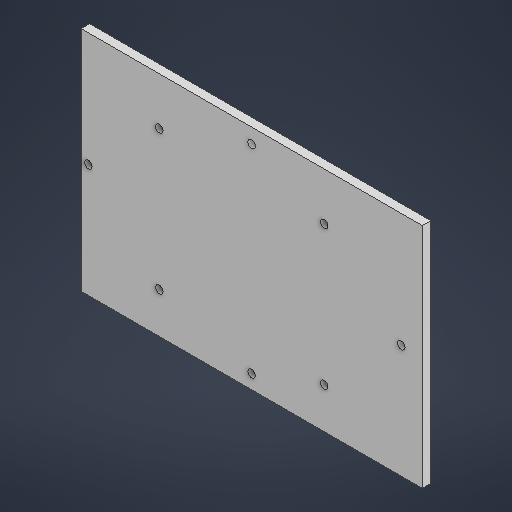
# Autodesk Inventor part: plate
Saved by Autodesk Inventor 2026.1 (Build 301233020, 233B)
## iProperties
Created: 2026-01-14
Part Number: plate
Material: Generic
Document SubType Name: Modeling
Designer: osama
Density: 1 g/cm^3
Appearance: Default
Author: osama
Autodesk Inventor part; units mm, degrees
ref_plane "YZ Plane" through (0, 0, 0) normal (1, 0, 0) x (0, 1, 0)
ref_plane "XZ Plane" through (0, 0, 0) normal (0, 1, 0) x (-1, 0, 0)
ref_plane "XY Plane" through (0, 0, 0) normal (0, 0, 1) x (1, 0, 0)
sketch "Sketch1" plane through (0, 0, 0) normal (0, 0, 1) x (1, 0, 0)
  line L0 (-60, -40) -> (60, -40)
  line L1 (60, -40) -> (60, 40)
  line L2 (60, 40) -> (-60, 40)
  line L3 (-60, 40) -> (-60, -40)
  line L4 (-60, -40) -> (60, 40) construction
  line L5 (60, -40) -> (-60, 40) construction
  line L6 (60, 0) -> (-60, 0)
  line L7 (0, -40) -> (0, 40)
  point P0 (0, 0)
  dimension "d0" = 120
  dimension "d1" = 80
  constraints: 16 end point, 6 midpoint, 2 parallel, 1 horizontal, 1 perpendicular
  measures "d0" distance of L2.end L1.end
  measures "d1" distance of L1.end L0.end
extrude "Extrusion1" add sketch "Sketch1" along normal blind 3
sketch "Sketch2" plane through (0, 0, 3) normal (0, 0, 1) x (1, 0, 0)
  circle A0 centre (-0.0328, 34.8037) radius 1.35
  circle A1 centre (-0.0328, -35.0463) radius 1.35
  circle A2 centre (52.5922, -0.1213) radius 1.35
  circle A3 centre (25.4936, 23.3086) radius 1.35
  circle A4 centre (25.4936, -25.6914) radius 1.35
  circle A5 centre (-32.5064, -25.6914) radius 1.35
  circle A6 centre (-32.5064, 23.3086) radius 1.35
  circle A7 centre (-57.4444, -0.1213) radius 1.35
  point P0 (0, 0)
  point P1 (-0.0328, -0.1213)
  constraints: 8 centre point
hole "Hole1" at (-0.0328, 34.8037, 3) at (-32.5064, 23.3086, 3) at (-57.4444, -0.1213, 3) at (-32.5064, -25.6914, 3) at (-0.0328, -35.0463, 3) at (25.4936, -25.6914, 3) at (52.5922, -0.1213, 3) at (25.4936, 23.3086, 3) direction (0, 0, -1) diameter 2.7 end through all
body "Solid1"
